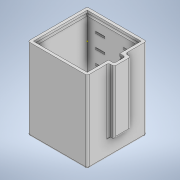
# Autodesk Inventor part: NEMA23_Shroud
Saved by Autodesk Inventor 2021 (Build 250183000, 183)
## iProperties
Created: 2021-03-31
Part Number: NEMA23_Shroud
Material: Generic
Document SubType Name: Modeling
Designer: Jorian Brusind
Density: 1 g/cm^3
Appearance: Default
Author: Jorian Brusind
Autodesk Inventor part; units mm, degrees
ref_plane "YZ Plane" through (0, 0, 0) normal (1, 0, 0) x (0, 1, 0)
ref_plane "XZ Plane" through (0, 0, 0) normal (0, 1, 0) x (-1, 0, 0)
ref_plane "XY Plane" through (0, 0, 0) normal (0, 0, 1) x (1, 0, 0)
ref_plane "Work Plane1" through (0, 3, 0) normal (0, 1, 0) x (1, 0, 0)
sketch "Sketch13" plane through (0, 0, 0) normal (0, 1, 0) x (-1, 0, 0)
  line L0 (-28.5, -28.5) -> (28.5, -28.5)
  line L1 (28.5, -28.5) -> (28.5, 28.5)
  line L2 (28.5, 28.5) -> (-28.5, 28.5)
  line L3 (-28.5, 28.5) -> (-28.5, -28.5)
  line L4 (-28.5, -28.5) -> (28.5, 28.5) construction
  line L5 (28.5, -28.5) -> (-28.5, 28.5) construction
  line L6 (-32, -32) -> (32, -32)
  line L7 (32, -32) -> (32, 32)
  line L8 (32, 32) -> (-32, 32)
  line L9 (-32, 32) -> (-32, -32)
  line L10 (-32, -32) -> (32, 32) construction
  line L11 (32, -32) -> (-32, 32) construction
  line L12 (-28.5, 28.5) -> (-32, 28.5)
  line L13 (-28.5, -28.5) -> (-32, -28.5)
  line L14 (-32, 29) -> (-32, 32)
  line L15 (-32, -31.5) -> (-32, -28.5)
  point P0 (0, 0)
  dimension "d117" = 57
  dimension "d118" = 57
  dimension "d119" = 64
  dimension "d120" = 64
  constraints: 32 end point, 4 midpoint, 4 parallel, 4 perpendicular, 2 horizontal, 2 point on line
  measures "d117" distance of L2.end L1.end
  measures "d118" distance of L1.end L0.end
  measures "d119" distance of L8.end L7.end
  measures "d120" distance of L7.end L6.end
extrude "Extrusion15" add sketch "Sketch13" along normal blind 3
sketch "Sketch19" plane through (0, 3, 0) normal (0, 1, 0) x (1, 0, 0)
  line L0 (-32, 32) -> (-32, -32) projected
  line L1 (32, 32) -> (-32, 32)
  line L2 (-32, 32) -> (-32, -32)
  line L3 (-32, -32) -> (32, -32)
  line L4 (32, -32) -> (32, 32)
  line L5 (32, 32) -> (-32, -32) construction
  line L6 (-32, 32) -> (32, -32) construction
  line L7 (29, 29) -> (-29, 29)
  line L8 (-29, 29) -> (-29, -29)
  line L9 (-29, -29) -> (29, -29)
  line L10 (29, -29) -> (29, 29)
  line L11 (29, 29) -> (-29, -29) construction
  line L12 (-29, 29) -> (29, -29) construction
  point P0 (0, 0)
  point P1 (-32, 32)
  dimension "d150" = 58
  dimension "d151" = 58
  constraints: 24 end point, 4 midpoint, 4 parallel, 2 horizontal, 2 perpendicular
  measures "d150" distance of L9.end L8.end
  measures "d151" distance of L8.end L7.end
extrude "Extrusion18" add sketch "Sketch19" along normal blind 85
sketch "Sketch20" plane through (0, 88, 0) normal (0, 1, 0) x (1, 0, 0)
  line L0 (26, 6) -> (32, 6)
  line L1 (32, 6) -> (32, -6)
  line L2 (32, -6) -> (26, -6)
  line L3 (26, -6) -> (26, 6)
  line L4 (29, 29) -> (29, -29) projected
  line L5 (26, 6) -> (32, -6) construction
  line L6 (32, 6) -> (26, -6) construction
  point P0 (0, 0)
  point P1 (29, 0)
  dimension "d154" = 6
  dimension "d155" = 12
  constraints: 12 end point, 3 midpoint, 2 parallel, 1 horizontal, 1 perpendicular
  measures "d154" distance of L1.end L2.end
  measures "d155" distance of L0.end L1.end
extrude "Extrusion19" cut sketch "Sketch20" against normal blind 62
sketch "Sketch21" plane through (0, 0, 0) normal (0, 0, 1) x (1, 0, 0)
  line L0 (-32, 88) -> (32, 88) projected
  line L1 (-32, 88) -> (-32, 84)
  line L2 (-32, 0) -> (-32, 88) projected
  line L3 (-32, 84) -> (-28.25, 84)
  line L4 (-28.25, 84) -> (-29.25, 84)
  line L5 (-29.25, 84) -> (-29.25, 85.5)
  ellipse E0 centre (-29.25, 84) end of major axis (-29.25, 85.5) minor radius 1
  point P0 (0, 0)
  dimension "d158" = 4
  dimension "d159" = 3.75
  dimension "d160" = 1
  dimension "d161" = 1.5
  constraints: 8 end point, 2 perpendicular, 2 point on line, 1 coincident, 1 vertical, 4 other
  measures "d158" distance of L0.start L1.end
  measures "d159" distance of L1.end L3.end
  measures "d160" distance of L3.end L4.end
  measures "d161" distance of L4.end L5.end
extrude "Extrusion20" cut sketch "Sketch21" against normal mid plane 58
sketch "Sketch22" plane through (0, 3, 0) normal (0, 1, 0) x (1, 0, 0)
  point P0 (0, 0)
pattern_circular "Circular Pattern1" count 4 over 360 about axis through (0, -10, 0) along (0, 1, 0) of "Extrusion20"
sketch "Sketch23" plane through (0, 3, 0) normal (0, 1, 0) x (1, 0, 0)
  line L0 (28, 28) -> (-28, 28)
  line L1 (-28, 28) -> (-28, -28)
  line L2 (-28, -28) -> (28, -28)
  line L3 (28, -28) -> (28, 28)
  line L4 (28, 28) -> (-28, -28) construction
  line L5 (-28, 28) -> (28, -28) construction
  line L6 (-28, -28) -> (-28, -23.4)
  line L7 (-28, -23.4) -> (-23.5, -23.4)
  line L8 (-28, -23.4) -> (-23.5, -23.4) construction
  circle A0 centre (-23.5, -23.4) radius 2.25
  circle A1 centre (-23.5, -23.4) radius 3.75
  point P0 (0, 0)
  dimension "d167" = 56
  dimension "d168" = 56
  dimension "d169" = 4.6
  dimension "d170" = 4.5
  dimension "d171" = 0
  dimension "d172" = 4.5
  dimension "d173" = 7.5
  constraints: 18 end point, 3 horizontal, 2 centre point, 2 coincident, 2 midpoint, 2 parallel, 1 collinear, 1 perpendicular, 1 point on line
  measures "d167" distance of L2.end L1.end
  measures "d168" distance of L1.end L0.end
  measures "d169" distance of L1.end L6.end
  measures "d170" distance of L6.end L7.end
  measures "d171" distance between parallel lines of L7 L8
  measures "d172" diameter of A0
  measures "d173" diameter of A1
extrude "Extrusion21" add sketch "Sketch23" along normal blind 13 contours A1
pattern_circular "Circular Pattern2" count 4 over 360 about axis through (0, -10, 0) along (0, 1, 0) of "Extrusion21"
sketch "Sketch24" plane through (0, 3, 0) normal (0, 1, 0) x (1, 0, 0)
  circle A0 centre (-23.5, -23.4) radius 2.25 projected
  circle A1 centre (-23.5, -23.4) radius 2.25
  point P0 (0, 0)
  dimension "d179" = 4.5
  constraints: 1 centre point, 1 coincident
  measures "d179" diameter of A1
extrude "Extrusion22" cut sketch "Sketch24" against normal through all
pattern_circular "Circular Pattern3" count 4 over 360 about axis through (0, -10, 0) along (0, 1, 0) of "Extrusion22"
sketch "Sketch25" plane through (0, 0, 0) normal (0, -1, 0) x (1, 0, 0)
  circle A0 centre (-23.5, 23.4) radius 2.25 projected
  circle A1 centre (-23.5, 23.4) radius 3.75
  circle A2 centre (-23.5, 23.4) radius 2.25
  point P0 (0, 0)
  dimension "d185" = 7.5
  constraints: 2 centre point, 2 coincident, 1 concentric
  measures "d185" diameter of A1
extrude "Extrusion23" cut sketch "Sketch25" against normal blind 2
fillet "Fillet2" radius 2 8 edges at (-32, 0, 0) (-32, 44, -32) (-32, 44, 32) (0, 0, -32) (0, 0, 32) (32, 44, -32) (32, 0, 0) (32, 44, 32)
fillet "Fillet3" radius 2 4 edges at (-23.4, 3, -27.25) (-27.25, 3, 23.4) (27.25, 3, -23.4) (23.4, 3, 27.25)
sketch "Sketch26" plane through (30, 2, -32) normal (0, 0, -1) x (-1, 0, 0)
  line L0 (60, 86) -> (0, 86) projected
  line L1 (30, 86) -> (30, 5.654)
  line L2 (-2, 0) -> (-2, 86) projected
  line L3 (-2, 0) -> (19.325, 0)
  line L4 (52.1952, 1) -> (8.2771, 1) projected
  line L5 (-2, 0) -> (19.325, 0) construction
  line L6 (19.325, 0) -> (19.325, 4.654)
  line L7 (19.325, 4.654) -> (33.625, 4.654)
  line L8 (33.625, 4.654) -> (33.625, 17.354)
  line L9 (33.625, 17.354) -> (19.325, 17.354)
  line L10 (19.325, 17.354) -> (19.325, 4.654)
  line L11 (34.625, 18.354) -> (34.625, 3.654)
  line L12 (34.625, 3.654) -> (18.325, 3.654)
  line L13 (18.325, 3.654) -> (18.325, 18.354)
  line L14 (18.325, 18.354) -> (34.625, 18.354)
  point P0 (30, -2)
  dimension "d190" = 80.346
  dimension "d191" = 21.325
  dimension "d192" = 0
  dimension "d193" = 14.3
  dimension "d194" = 12.7
  dimension "d195" = 1
  constraints: 24 end point, 5 parallel, 3 perpendicular, 2 horizontal, 1 collinear, 1 midpoint, 1 vertical, 3 other
  measures "d190" distance of L1.start L1.end
  measures "d191" distance of L2.start L3.end
  measures "d192" distance between parallel lines of L3 L5
  measures "d193" distance of L9.end L8.end
  measures "d194" distance of L8.end L7.end
  measures "d195" distance between parallel lines of L8 L11
extrude "Extrusion24" cut sketch "Sketch26" against normal blind 3
fillet "Fillet4" radius 2 4 edges at (-4.625, 13.004, -32) (3.525, 5.654, -32) (11.675, 13.004, -32) (3.525, 20.354, -32)
fillet "Fillet5" radius 2 1 edges at (32, 26, 0)
pattern_circular "Circular Pattern4" count 4 over 360 about axis through (0, -10, 0) along (0, 1, 0) of "Extrusion23"
sketch "Sketch27" plane through (0, 88, 0) normal (0, 1, 0) x (1, 0, 0)
  point P0 (0, 0)
sketch "Sketch28" plane through (0, 88, 0) normal (0, 1, 0) x (1, 0, 0)
  line L0 (32, -30) -> (32, -6) projected
  line L1 (32, -6) -> (35, -6)
  line L2 (35, -6) -> (35, 6)
  line L3 (35, 6) -> (32, 6)
  line L4 (32, 6) -> (32, -6)
  line L5 (38, 9) -> (38, -9)
  line L6 (38, -9) -> (29, -9)
  line L7 (29, 9) -> (38, 9)
  line L8 (32, -6) -> (32, -9)
  line L9 (32, 6) -> (32, 9)
  line L10 (32, 30) -> (32, -30) projected
  point P0 (0, 0)
  point P1 (32, -9)
  dimension "d204" = 3
  dimension "d205" = 12
  dimension "d206" = 3
  dimension "d207" = 3
  dimension "d208" = 9
  dimension "d209" = 3
  constraints: 18 end point, 3 parallel, 3 point on line, 2 perpendicular, 1 horizontal, 1 other
  measures "d204" distance of L3.end L2.end
  measures "d205" distance of L2.end L1.end
  measures "d206" distance between parallel lines of L2 L5
  measures "d207" distance of L0.end L8.end
  measures "d208" distance of L7.start L5.start
  measures "d209" distance between parallel lines of L3 L7
extrude "Extrusion25" add sketch "Sketch28" against normal blind 68 contours L0 L1 L2 L3 L9 L7 L5 L6
sketch "Sketch29" plane through (0, 20, 0) normal (0, -1, 0) x (1, 0, 0)
  line L0 (38, 9) -> (38, -9) projected
  line L1 (32, -9) -> (38, -9) projected
  line L2 (38, 9) -> (32, 9)
  line L3 (32, 9) -> (32, -9)
  line L4 (32, -9) -> (38, -9)
  line L5 (38, -9) -> (38, 9)
  point P0 (0, 0)
  constraints: 8 end point, 2 parallel, 1 horizontal, 1 perpendicular
extrude "Extrusion26" add sketch "Sketch29" against normal blind 3
fillet "Fillet7" radius 2 6 edges at (38, 54, 9) (32, 54, 9) (32, 20, 0) (38, 20, 0) (32, 54, -9) (38, 54, -9)
fillet "Fillet8" radius 2 2 edges at (35, 55.5, 6) (35, 55.5, -6)
fillet "Fillet9" radius 2 5 edges at (34.4142, 23, 5.4142) (32.5, 23, 6) (34.4142, 23, -5.4142) (32.5, 23, -6) (35, 23, 0)
sketch "Sketch30" plane through (30, 2, -32) normal (0, 0, -1) x (-1, 0, 0)
  line L0 (10, 71) -> (20, 71)
  line L1 (20, 71) -> (20, 69)
  line L2 (20, 69) -> (10, 69)
  line L3 (10, 69) -> (10, 71)
  line L4 (0, 86) -> (60, 86) projected
  line L5 (0, 0) -> (0, 86) projected
  line L6 (40, 71) -> (50, 71)
  line L7 (50, 71) -> (50, 69)
  line L8 (50, 69) -> (40, 69)
  line L9 (40, 69) -> (40, 71)
  line L10 (10, 56) -> (20, 56)
  line L11 (20, 56) -> (20, 54)
  line L12 (20, 54) -> (10, 54)
  line L13 (10, 54) -> (10, 56)
  line L14 (40, 56) -> (50, 56)
  line L15 (50, 56) -> (50, 54)
  line L16 (50, 54) -> (40, 54)
  line L17 (40, 54) -> (40, 56)
  line L18 (10, 41) -> (20, 41)
  line L19 (20, 41) -> (20, 39)
  line L20 (20, 39) -> (10, 39)
  line L21 (10, 39) -> (10, 41)
  line L22 (40, 41) -> (50, 41)
  line L23 (50, 41) -> (50, 39)
  line L24 (50, 39) -> (40, 39)
  line L25 (40, 39) -> (40, 41)
  point P0 (30, -2)
  dimension "d217" = 10
  dimension "d218" = 2
  dimension "d219" = 15
  dimension "d220" = 10
  dimension "d223" = 30
  dimension "d226" = 15
  constraints: 48 end point, 2 horizontal, 2 parallel, 1 perpendicular, 1 vertical, 40 other
  measures "d217" distance of L1.end L2.end
  measures "d218" distance of L0.end L1.end
  measures "d219" distance between parallel lines of L4 L0
  measures "d220" distance between parallel lines of L5 L3
  measures "d223" distance of L0.start L6.start
  measures "d226" distance of L0.start L10.start
extrude "Extrusion27" cut sketch "Sketch30" against normal blind 3
sketch "Sketch2" plane through (0, 3, 0) normal (0, 1, 0) x (1, 0, 0)
  line L0 (0, 12.2943) -> (0, 43.7057)
  arc A0 (-3.0277, 9.4339) -> (0, 12.2943) centre (-2.9968, 12.4338) ccw
  line L1 (-4.5807, 9.4339) -> (-3.0277, 9.4339)
  arc A1 (-4.5807, 9.4339) -> (-9.0279, 4.4646) centre (-4.0279, 4.4646) ccw
  line L2 (-9.0279, 2.9638) -> (-9.0279, 4.4646)
  arc A2 (-12.0277, 0) -> (-9.0279, 2.9638) centre (-12.0277, 3) ccw
  line L3 (-44.022, 0) -> (-12.0277, 0)
  arc A3 (-46.5576, 2.9638) -> (-44.022, 0) centre (-43.5576, 2.9638) ccw
  line L4 (-46.5576, 4.5169) -> (-46.5576, 2.9638)
  arc A4 (-46.5576, 4.5169) -> (-51.5269, 8.9638) centre (-51.5269, 3.9638) ccw
  line L5 (-53.0277, 8.9638) -> (-51.5269, 8.9638)
  arc A5 (-56, 11.5573) -> (-53.0277, 8.9638) centre (-53.0277, 11.9638) ccw
  line L6 (-56, 44.3704) -> (-56, 11.5573)
  arc A6 (-53.0277, 46.9638) -> (-56, 44.3704) centre (-53.0277, 43.9638) ccw
  arc A7 (-51.5269, 46.9638) -> (-46.5576, 51.4108) centre (-51.5269, 51.9638) ccw
  line L7 (-51.5269, 46.9638) -> (-53.0277, 46.9638)
  arc A8 (-43.5578, 56) -> (-46.5576, 52.9638) centre (-43.5578, 53) ccw
  line L8 (-46.5576, 52.9638) -> (-46.5576, 51.4108)
  line L9 (-12.0277, 56) -> (-43.5578, 56)
  arc A9 (-9.0277, 53) -> (-12.0277, 56) centre (-12.0277, 53) ccw
  line L10 (-9.0277, 51.4993) -> (-9.0277, 53)
  arc A10 (-9.0277, 51.4993) -> (-4.5807, 46.5299) centre (-4.0277, 51.4993) ccw
  line L11 (-3.0277, 46.5299) -> (-4.5807, 46.5299)
  arc A11 (0, 43.7057) -> (-3.0277, 46.5299) centre (-2.9949, 43.5301) ccw
  arc A12 (-43.5578, 58) -> (-48.5576, 52.9533) centre (-43.5578, 53) ccw
  line L12 (-48.5576, 52.9533) -> (-48.5576, 51.5359)
  arc A13 (-51.5269, 48.9638) -> (-48.5576, 51.5359) centre (-51.5269, 51.9638) ccw
  line L13 (-51.5269, 48.9638) -> (-53.0277, 48.9638)
  arc A14 (-53.0277, 48.9638) -> (-58, 44.4892) centre (-53.0277, 43.9638) ccw
  line L14 (-58, 44.4892) -> (-58, 11.4385)
  arc A15 (-58, 11.4385) -> (-53.0277, 6.9638) centre (-53.0277, 11.9638) ccw
  line L15 (-53.0277, 6.9638) -> (-51.5269, 6.9638)
  arc A16 (-48.5576, 4.3918) -> (-51.5269, 6.9638) centre (-51.5269, 3.9638) ccw
  line L16 (-48.5576, 4.3918) -> (-48.5576, 2.9638)
  arc A17 (-48.5576, 2.9638) -> (-44.1579, -2) centre (-43.5576, 2.9638) ccw
  line L17 (-44.1579, -2) -> (-12.0277, -2)
  arc A18 (-12.0277, -2) -> (-7.0279, 2.9533) centre (-12.0277, 3) ccw
  line L18 (-7.0279, 2.9533) -> (-7.0279, 4.4646)
  arc A19 (-4.4557, 7.4339) -> (-7.0279, 4.4646) centre (-4.0279, 4.4646) ccw
  line L19 (-4.4557, 7.4339) -> (-3.0367, 7.4339)
  arc A20 (-3.0367, 7.4339) -> (2, 12.2537) centre (-2.9968, 12.4338) ccw
  line L20 (2, 12.2537) -> (2, 43.7568)
  arc A21 (2, 43.7568) -> (-3.0372, 48.5299) centre (-2.9949, 43.5301) ccw
  line L21 (-3.0372, 48.5299) -> (-4.4556, 48.5299)
  arc A22 (-7.0277, 51.4993) -> (-4.4556, 48.5299) centre (-4.0277, 51.4993) ccw
  line L22 (-7.0277, 51.4993) -> (-7.0277, 53)
  arc A23 (-7.0277, 53) -> (-12.0277, 58) centre (-12.0277, 53) ccw
  line L23 (-12.0277, 58) -> (-43.5578, 58)
  line L24 (0, 0) -> (-56, 0)
  line L25 (0, 0) -> (0, 56)
  dimension "d17" = 5
  dimension "d18" = 5
  dimension "d19" = 5
  dimension "d20" = 5
  dimension "d24" = 2
  dimension "d28" = 56
  dimension "d29" = 56
  constraints: 52 end point, 48 point on circle, 24 centre point, 2 point on line, 23 other
  measures "d17" radius of A7
  measures "d18" radius of A4
  measures "d19" radius of A1
  measures "d20" radius of A10
  measures "d24" distance between parallel lines of L9 L23
  measures "d28" distance of L24.start L24.end
  measures "d29" distance of L24.start L25.end
sketch "Sketch3" plane through (0, 3, 0) normal (0, -1, 0) x (1, 0, 0)
  line L0 (0, -43.7057) -> (0, -12.2943) projected
  line L1 (0, -12.2943) -> (0, -43.7057)
  line L2 (-43.5578, -56) -> (-12.0277, -56) projected
  arc A0 (-12.0277, -56) -> (-9.0277, -53) centre (-12.0277, -53) ccw projected
  arc A1 (-4.5807, -46.5299) -> (-9.0277, -51.4993) centre (-4.0277, -51.4993) ccw projected
  line L3 (-9.0277, -53) -> (-9.0277, -51.4993) projected
  arc A2 (-3.0277, -46.5299) -> (0, -43.7057) centre (-2.9949, -43.5301) ccw projected
  line L4 (-4.5807, -46.5299) -> (-3.0277, -46.5299) projected
  arc A3 (-46.5576, -52.9638) -> (-43.5578, -56) centre (-43.5578, -53) ccw projected
  arc A4 (-46.5576, -51.4108) -> (-51.5269, -46.9638) centre (-51.5269, -51.9638) ccw projected
  line L5 (-46.5576, -51.4108) -> (-46.5576, -52.9638) projected
  arc A5 (-56, -44.3704) -> (-53.0277, -46.9638) centre (-53.0277, -43.9638) ccw projected
  line L6 (-53.0277, -46.9638) -> (-51.5269, -46.9638) projected
  line L7 (-56, -11.5573) -> (-56, -44.3704) projected
  arc A6 (-53.0277, -8.9638) -> (-56, -11.5573) centre (-53.0277, -11.9638) ccw projected
  line L8 (-51.5269, -8.9638) -> (-53.0277, -8.9638) projected
  arc A7 (-51.5269, -8.9638) -> (-46.5576, -4.5169) centre (-51.5269, -3.9638) ccw projected
  arc A8 (-44.022, 0) -> (-46.5576, -2.9638) centre (-43.5576, -2.9638) ccw projected
  line L9 (-12.0277, 0) -> (-44.022, 0) projected
  line L10 (-46.5576, -2.9638) -> (-46.5576, -4.5169) projected
  arc A9 (-9.0279, -2.9638) -> (-12.0277, 0) centre (-12.0277, -3) ccw projected
  line L11 (-9.0279, -4.4646) -> (-9.0279, -2.9638) projected
  arc A10 (-9.0279, -4.4646) -> (-4.5807, -9.4339) centre (-4.0279, -4.4646) ccw projected
  line L12 (-3.0277, -9.4339) -> (-4.5807, -9.4339) projected
  arc A11 (0, -12.2943) -> (-3.0277, -9.4339) centre (-2.9968, -12.4338) ccw projected
  point P0 (0, 0)
  constraints: 2 end point, 1 collinear
sketch "Sketch4" plane through (0, 77, 0) normal (0, 1, 0) x (1, 0, 0)
  line L0 (2, 12.2537) -> (2, 43.7568) projected
  line L1 (2, 28.0053) -> (-58, 27.9638)
  line L2 (-58, 44.4892) -> (-58, 11.4385) projected
  line L3 (-12.0277, 58) -> (-43.5578, 58) projected
  line L4 (-27.7928, 58) -> (-28.0928, -2)
  line L5 (-44.1579, -2) -> (-12.0277, -2) projected
  line L6 (2.0572, 58) -> (-57.9428, 58)
  line L7 (-57.9428, 58) -> (-57.9428, -2)
  line L8 (-57.9428, -2) -> (2.0572, -2)
  line L9 (2.0572, -2) -> (2.0572, 58)
  line L10 (2.0572, 58) -> (-57.9428, -2) construction
  line L11 (-57.9428, 58) -> (2.0572, -2) construction
  arc A0 (-4.4557, 7.4339) -> (-7.0279, 4.4646) centre (-4.0279, 4.4646) ccw projected
  line L12 (-7.0279, 2.9533) -> (-7.0279, 4.4646) projected
  arc A1 (-12.0277, -2) -> (-7.0279, 2.9533) centre (-12.0277, 3) ccw projected
  arc A2 (-3.0367, 7.4339) -> (2, 12.2537) centre (-2.9968, 12.4338) ccw projected
  line L13 (-4.4557, 7.4339) -> (-3.0367, 7.4339) projected
  arc A3 (2, 43.7568) -> (-3.0372, 48.5299) centre (-2.9949, 43.5301) ccw projected
  line L14 (-3.0372, 48.5299) -> (-4.4556, 48.5299) projected
  arc A4 (-7.0277, 51.4993) -> (-4.4556, 48.5299) centre (-4.0277, 51.4993) ccw projected
  line L15 (-7.0277, 51.4993) -> (-7.0277, 53) projected
  arc A5 (-7.0277, 53) -> (-12.0277, 58) centre (-12.0277, 53) ccw projected
  arc A6 (-43.5578, 58) -> (-48.5576, 52.9533) centre (-43.5578, 53) ccw projected
  line L16 (-48.5576, 52.9533) -> (-48.5576, 51.5359) projected
  arc A7 (-51.5269, 48.9638) -> (-48.5576, 51.5359) centre (-51.5269, 51.9638) ccw projected
  line L17 (-51.5269, 48.9638) -> (-53.0277, 48.9638) projected
  arc A8 (-53.0277, 48.9638) -> (-58, 44.4892) centre (-53.0277, 43.9638) ccw projected
  arc A9 (-58, 11.4385) -> (-53.0277, 6.9638) centre (-53.0277, 11.9638) ccw projected
  line L18 (-53.0277, 6.9638) -> (-51.5269, 6.9638) projected
  arc A10 (-48.5576, 4.3918) -> (-51.5269, 6.9638) centre (-51.5269, 3.9638) ccw projected
  line L19 (-48.5576, 4.3918) -> (-48.5576, 2.9638) projected
  arc A11 (-48.5576, 2.9638) -> (-44.1579, -2) centre (-43.5576, 2.9638) ccw projected
  point P0 (0, 0)
  point P1 (-27.9428, 28)
  point P2 (-57.9428, 44.8814)
  point P3 (-57.9428, 11.0463)
  point P4 (-44.1579, -2)
  dimension "d64" = 60
  dimension "d65" = 60
  constraints: 16 end point, 7 midpoint, 2 parallel, 1 horizontal, 1 perpendicular
  measures "d64" distance of L8.end L7.end
  measures "d65" distance of L7.end L6.end
sketch "Sketch7" plane through (0, 73, 0) normal (0, -1, 0) x (1, 0, 0)
  circle A0 centre (-4.5, -4.5) radius 2.75
  line L0 (-12.0277, 0) -> (-44.022, 0) projected
  line L1 (0, -43.7057) -> (0, -12.2943) projected
  line L2 (-44.022, 0) -> (-12.0277, 0)
  line L3 (-56, -11.5573) -> (-56, -44.3704) projected
  line L4 (-56, -11.5573) -> (-56, -44.3704)
  circle A1 centre (-51.5, -4.5) radius 2.75
  circle A2 centre (-4.5, -51.5) radius 2.75
  circle A3 centre (-51.5, -51.5) radius 2.75
  point P0 (0, 0)
  dimension "d68" = 5.5
  dimension "d69" = 4.5
  dimension "d70" = 4.5
  dimension "d73" = 47
  dimension "d76" = 47
  constraints: 4 centre point, 4 end point, 2 vertical, 1 collinear, 1 horizontal, 6 other
  measures "d68" diameter of A0
  measures "d69" distance from line of L0 A0.centre
  measures "d70" distance from line of L1 A0.centre
  measures "d73" distance of A0.centre A1.centre
  measures "d76" distance of A0.centre A2.centre
sketch "Sketch8" plane through (0, 73, 0) normal (0, -1, 0) x (1, 0, 0)
  circle A0 centre (-51.5, -4.5) radius 2.75 projected
  circle A1 centre (-51.5, -4.5) radius 0.5
  circle A2 centre (-51.5, -4.5) radius 5.5
  line L0 (-44.1579, 2) -> (-57.9428, 2) projected
  line L1 (-57.9428, 2) -> (-44.1579, 2)
  line L2 (-58, -44.4892) -> (-58, -11.4385) projected
  line L3 (-57.9428, 2) -> (-58, -11.4385)
  circle A3 centre (-4.5, -4.5) radius 0.5
  circle A4 centre (-4.5, -4.5) radius 5.5
  circle A5 centre (-51.7002, -51.4996) radius 0.5
  circle A6 centre (-51.7002, -51.4996) radius 5.5
  circle A7 centre (-4.7002, -51.4996) radius 0.5
  circle A8 centre (-4.7002, -51.4996) radius 5.5
  point P0 (0, 0)
  dimension "d81" = 1
  dimension "d82" = 11
  dimension "d85" = 47
  dimension "d88" = 47
  constraints: 8 centre point, 5 coincident, 4 end point, 1 collinear, 1 horizontal, 13 other
  measures "d81" diameter of A1
  measures "d82" diameter of A2
  measures "d85" distance of A1.centre A3.centre
  measures "d88" distance of A1.centre A5.centre
sketch "Sketch9" plane through (0, 73, 0) normal (0, -1, 0) x (1, 0, 0)
  circle A0 centre (-51.5, -4.5) radius 2.75 projected
  circle A1 centre (-51.5, -4.5) radius 3.5
  point P0 (0, 0)
  dimension "d93" = 7
  dimension "d96" = 1
  dimension "d97" = 2
  dimension "d98" = 2
  dimension "d99" = 64
  dimension "d100" = 64
  constraints: 22 end point, 4 parallel, 3 perpendicular, 2 horizontal, 2 vertical, 1 midpoint
sketch "Sketch11" plane through (-58, 3, -44.4892) normal (-1, 0, 0) x (0, 0, 1)
  line L0 (0.7835, 74) -> (32.1949, 74) projected
  line L1 (16.4892, 74) -> (89.1352, 74) construction
  line L2 (-11.5108, 3) -> (-11.5108, 74) projected
  line L3 (-11.5108, 74) -> (5.3542, 74)
  line L4 (0, 74) -> (33.0508, 74) projected
  line L5 (-11.5108, 74) -> (5.3542, 74) construction
  line L6 (5.3542, 74) -> (5.3542, 16.854)
  line L7 (5.3542, 74) -> (62.5002, 74) construction
  line L8 (5.3542, 16.854) -> (21.6542, 16.854)
  line L9 (21.6542, 16.854) -> (21.6542, 3.154)
  line L10 (21.6542, 3.154) -> (5.3542, 3.154)
  line L11 (5.3542, 3.154) -> (5.3542, 16.854)
  point P0 (44.4892, -3)
  dimension "d103" = 16.865
  dimension "d104" = 0
  dimension "d105" = 57.146
  dimension "d106" = 90
  dimension "d107" = 16.3
  dimension "d108" = 13.7
  constraints: 18 end point, 4 horizontal, 2 equal length, 2 parallel, 1 collinear, 1 midpoint, 1 perpendicular, 1 vertical
  measures "d103" distance of L2.end L3.end
  measures "d104" distance between parallel lines of L5 L3
  measures "d105" distance of L5.end L6.end
  measures "d106" angle of L6 L7
  measures "d107" distance of L9.end L10.end
  measures "d108" distance of L8.end L9.end
sketch "Sketch12" plane through (-12.0277, 3, -58) normal (0, 0, -1) x (-1, 0, 0)
  line L0 (-14.0849, 74) -> (-14.0849, 70) projected
  line L1 (-14.0849, 74) -> (5.4631, 74)
  line L2 (0, 74) -> (31.9943, 74) projected
  line L3 (5.4631, 74) -> (5.4631, 65)
  circle A0 centre (5.4631, 65) radius 1.5
  point P0 (-12.0277, -3)
  dimension "d111" = 19.548
  dimension "d112" = 9
  dimension "d113" = 3
  constraints: 4 end point, 1 centre point, 1 coincident, 1 point on line, 1 vertical
  measures "d111" distance of L0.start L1.end
  measures "d112" distance of L1.end L3.end
  measures "d113" diameter of A0
body "Solid1"
body "Solid3"
